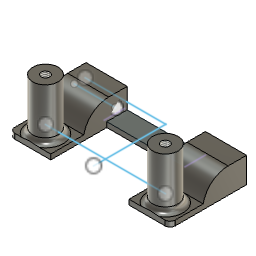
Bela_blocker (Autodesk Fusion 360 design; units mm, degrees)
Autodesk Fusion 360 part; units mm, degrees
note: some values were not read from the file. Chosen so that the rebuilt part matches the saved one: which face or edge a step refers to. Set by a fixed rule: which sketch regions a step uses.
sketch "Sketch1" plane through (0, 0, 0) normal (0, 0, 1) x (1, 0, 0)
  line L0 (-26.5, -4) -> (26.5, -4)
  line L1 (26.5, -4) -> (26.5, 4)
  line L2 (26.5, 4) -> (-26.5, 4)
  line L3 (-26.5, 4) -> (-26.5, -4)
  line L4 (-26.5, -4) -> (26.5, 4) construction
  line L5 (26.5, -4) -> (-26.5, 4) construction
  dimension "d1" = 53
  dimension "d2" = 8
  constraint horizontal L0
  constraint perpendicular L0 L1
  constraint parallel L0 L2
  constraint parallel L1 L3
  constraint coincident L4 origin
  constraint coincident L5 origin
  measures "d1" distance of L1.end L2.end
  measures "d2" distance of L0.end L1.end
extrude "Extrude1" add sketch "Sketch1" along normal blind 2
sketch "Sketch2" plane through (0, 0, 2) normal (0, 0, 1) x (-1, 0, 0)
  line L0 (26.5, -4) -> (26.5, 4)
  line L1 (26.5, 4) -> (-26.5, 4)
  line L2 (-26.5, 4) -> (-26.5, -4)
  line L3 (-26.5, -4) -> (26.5, -4)
  circle A0 centre (0, 0) radius 1.5
  dimension "d7" = 3
  constraint coincident A0.centre origin
  measures "d7" diameter of A0
extrude "Extrude2" cut sketch "Sketch2" against normal blind 2 contours A0
move_face "MoveFace1" to x (1, 0, 0) y (0, 1, 0) z (0, 0, 1) at (-22.25, 0, 0) 1 faces at (-1.4925, 0.1494, 0.6667)
sketch "Sketch3" plane through (0, 0, 2) normal (0, 0, 1) x (-1, 0, 0)
  circle A0 centre (22.25, 0) radius 1.5
  line L0 (26.5, -4) -> (26.5, 4)
  line L1 (26.5, 4) -> (-26.5, 4)
  line L2 (-26.5, 4) -> (-26.5, -4)
  line L3 (-26.5, -4) -> (26.5, -4)
  circle A1 centre (0, 0) radius 1.5
  dimension "d10" = 3
  constraint coincident A1.centre origin
  measures "d10" diameter of A1
extrude "Extrude3" cut sketch "Sketch3" against normal blind 2 contours A1
move_face "MoveFace2" to x (1, 0, 0) y (0, 1, 0) z (0, 0, 1) at (22.25, 0, 0) 1 faces at (-1.4925, 0.1494, 0.6667)
extrude "Extrude4" add 1 faces at (8.8333, 4, 0.6667) along direction (0, 1, 0) blind 20
sketch "Sketch4" plane through (0, -4, 0) normal (0, -1, 0) x (1, 0, 0)
  line L0 (-26.5, 0) -> (26.5, 0)
  line L1 (26.5, 2) -> (-26.5, 2)
  line L2 (-26.5, 0) -> (-19.5, 0)
  line L3 (26.5, 0) -> (20.5, 0)
  line L4 (-19.5, 0) -> (-19.5, 2)
  line L5 (20.5, 0) -> (20.5, 2)
  line L6 (26.5, 0) -> (26.5, 2)
  line L7 (-26.5, 2) -> (-26.5, 0)
  dimension "d21" = 6
  constraint coincident L0.start L2.start
  constraint coincident L0 L2.end
  constraint coincident L0.end L3.start
  constraint coincident L0 L3.end
  constraint coincident L1 L4.end
  constraint perpendicular L1 L4
  constraint coincident L1 L5.end
  constraint perpendicular L1 L5
  measures "d21" distance of L0.end L3.end
extrude "Extrude5" cut sketch "Sketch4" against normal blind 20 contours L0 L1 L4 L5
sketch "Sketch5" plane through (0, 0, 0) normal (0, 0, -1) x (1, 0, 0)
  line L0 (20.5, 4) -> (20.5, -16)
  line L1 (20.5, -16) -> (-19.5, -16)
  line L2 (-19.5, -16) -> (-19.5, 4)
  line L3 (-19.5, 4) -> (-26.5, 4)
  line L4 (-26.5, 4) -> (-26.5, -24)
  line L5 (-26.5, -24) -> (26.5, -24)
  line L6 (26.5, -24) -> (26.5, 4)
  circle A0 centre (22.25, 0) radius 1.5
  circle A1 centre (-22.25, 0) radius 1.5
  line L7 (20.5, -16) -> (20.5, -24)
  line L8 (-19.5, -16) -> (-19.5, -24)
  line L9 (20.5, -4.9584) -> (26.5, -4.9584)
  line L10 (-19.5, -4.9584) -> (-26.5, -4.9584)
  line L11 (26.5, 4) -> (20.5, 4)
  constraint coincident L0.end L1.start
  constraint coincident L5 L7.end
  constraint perpendicular L5 L7
  constraint coincident L1.end L2.start
  constraint coincident L5 L8.end
  constraint perpendicular L5 L8
  constraint coincident L0 L9.start
  constraint coincident L6 L9.end
  constraint perpendicular L6 L9
  constraint coincident L2 L10.start
  constraint coincident L4 L10.end
  constraint perpendicular L4 L10
extrude "Extrude6" add sketch "Sketch5" along normal blind 5 contours L0 L5 L6 L7 L9 | L2 L4 L5 L8 L10
extrude "Extrude7" add 1 faces at (20.5, 14.9861, -3.3333) along direction (-1, 0, 0) blind 4.45
extrude "Extrude8" add 1 faces at (-19.5, 14.9861, -3.3333) along direction (1, 0, 0) blind 4.45
move_body "Move1" bodies 1 to x (-1, 0, 0) y (0, 1, 0) z (0, 0, -1) at (-30.1, 0, -3)
extrude "Extrude9" cut 1 faces at (-46.15, 14.9861, 0.3333) along direction (-1, 0, 0) blind 0.3
extrude "Extrude10" cut 1 faces at (-15.05, 14.9861, 0.3333) along direction (1, 0, 0) blind 0.3
extrude "Extrude11" add 2 faces at (-53.2167, 11.3056, 2) (-7.3167, 11.3056, 2) along direction (0, 0, 1) blind 3
sketch "Sketch6" plane through (0, 0, -3) normal (0, 0, 1) x (1, 0, 0)
  line L0 (-14.75, 24) -> (-46.45, 24)
  line L1 (-46.45, 16) -> (-14.75, 16)
  line L2 (-46.45, 24) -> (-46.45, 16)
  line L3 (-14.75, 16) -> (-14.75, 24)
sketch "Sketch7" plane through (0, -4, 0) normal (0, -1, 0) x (1, 0, 0)
  line L0 (-14.75, -3) -> (-14.75, -5)
  line L1 (-14.75, -5) -> (-3.6, -5)
  line L2 (-3.6, -3) -> (-14.75, -3)
  line L3 (-3.6, -5) -> (-3.6, -3)
sketch "Sketch8" plane through (-3.6, 0, 0) normal (1, 0, 0) x (0, 1, 0)
  line L0 (4.9584, -3) -> (-4, -3)
  line L1 (-4, -3) -> (-4, -5)
  line L2 (-4, -5) -> (24, -5)
  line L3 (24, -5) -> (24, 5)
  line L4 (24, 5) -> (4.9584, 5)
  line L5 (4.9584, 5) -> (4.9584, -3)
extrude "Extrude12" add sketch "Sketch8" along normal blind 5
extrude "Extrude13" add 1 faces at (-56.6, 17.6528, -1) along direction (-1, 0, 0) blind 5
sketch "Sketch9" plane through (0, 0, 0) normal (0, 0, 1) x (1, 0, 0)
  line L0 (-61.5981, 23.6667) -> (-30, 23.6667)
  line L1 (-30, 23.6667) -> (-30, -4.5955)
  line L2 (-30, 0) -> (-6.5, 0)
  line L3 (-30, 0) -> (-53.5, 0)
  dimension "d49" = 23.5
  dimension "d50" = 23.5
  constraint horizontal L0
  constraint horizontal L2
  constraint coincident L1 L2.start
  constraint perpendicular L1 L3
  measures "d49" distance of L2.start L2.end
  measures "d50" distance of L2.start L3.end
move_face "MoveFace3" to x (1, 0, 0) y (0, 1, 0) z (0, 0, 1) at (-1.1462, -0.0121, 0) 1 faces at (-51.9437, -1.4439, -3.6667)
move_face "MoveFace4" to x (1, 0, 0) y (0, 1, 0) z (0, 0, 1) at (1.3656, 0, 0) 1 faces at (-6.3575, 0.1494, -4.3333)
fillet "Fillet9" radius 2 1 edges at (1.4, -4, -4)
sketch "Sketch10" plane through (0, 0, 0) normal (0, 0, 1) x (1, 0, 0)
extrude "Extrude14" add 1 faces at (-46.45, 14.9861, 2.3333) along direction (1, 0, 0) blind 1
sketch "Sketch11" plane through (0, 0, 0) normal (0, 0, 1) x (1, 0, 0)
  line L0 (-61.676, 19.4601) -> (-45.5115, 19.4601)
  constraint horizontal L0
sketch "Sketch12" plane through (0, 0, -3) normal (0, 0, 1) x (-1, 0, 0)
  line L0 (14.75, -4.9584) -> (14.75, 4)
  arc A0 (0.6, 4) -> (-1.4, 2) centre (0.6, 2) ccw
  line L1 (-1.4, 2) -> (-1.4, -4.9584)
  circle A1 centre (6.4844, 0) radius 1.5
  circle A2 centre (6.4844, 0) radius 5
  dimension "d65" = 10
  constraint concentric A1 A2
  measures "d65" diameter of A2
extrude "Extrude15" add sketch "Sketch7" along normal blind 2
delete_face "DeleteFace8" 1 faces at (-0.4099, -3.9909, -4.3333)
extrude "Extrude16" add 1 faces at (-1.9333, -4, -3.6667) along direction (0, -1, 0) blind 2
sketch "Sketch13" plane through (0, 0, -3) normal (0, 0, 1) x (-1, 0, 0)
  line L0 (61.6, -4.9584) -> (61.6, 4)
  line L1 (45.45, 4) -> (45.45, -4.9584)
  circle A0 centre (53.4962, 0.0121) radius 1.5
  circle A1 centre (53.4962, 0.0121) radius 5
  dimension "d70" = 10
  constraint concentric A0 A1
  measures "d70" diameter of A1
extrude "Extrude17" add 1 faces at (-56.2167, -4, -4.3333) along direction (0, -1, 0) blind 2
fillet "Fillet15" radius 2 2 edges at (-61.6, -6, -4) (1.4, -6, -4)
delete_face "DeleteFace11" 1 faces at (-61.5909, -4.1901, -3.6667)
delete_face "DeleteFace12" 1 faces at (-0.5048, -5.9977, -4.3333)
extrude "Extrude18" cut 1 faces at (-50.8333, 4.9584, 2.3333) along direction (0, 1, 0) blind 2
extrude "Extrude19" add sketch "Sketch13" along normal blind 20
extrude "Extrude20" cut 1 faces at (-3.9833, 4.9584, 2.3333) along direction (0, 1, 0) blind 2
extrude "Extrude21" add sketch "Sketch12" along normal blind 20
delete_face "DeleteFace13" 2 faces at (-51.9981, 0.0627, -3.6667) (-54.9887, 0.1373, 3.6667)
delete_face "DeleteFace14" 2 faces at (-7.977, 0.1494, 3.6667) (-4.9863, 0.0748, -3.6667)
hole "Hole1" at (-6.4844, 0, 17) direction (0, 0, -1) diameter 3.332 depth 10 tip angle 118
thread "Thread1" "ISO Metric profile 4.0 M4x0.7 6H"
hole "Hole2" at (-53.4962, -0.0121, 17) direction (0, 0, -1) diameter 3.332 depth 10 tip angle 118
thread "Thread2" "ISO Metric profile 4.0 M4x0.7 6H"
fillet "Fillet16" radius 10 2 edges at (-53.525, 6.9584, 5) (-6.675, 6.9584, 5)
fillet "Fillet17" radius 2 1 edges at (-48.8346, -1.8201, -3)
fillet "Fillet18" radius 2 1 edges at (-1.8228, -1.8081, -3)
fillet "Fillet19" radius 2 2 edges at (-61.6, -6, -4) (1.4, -6, -4)
